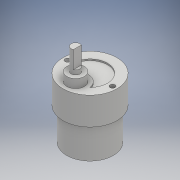
# Autodesk Inventor part: MOTOR DC
Saved by Autodesk Inventor 2018 (Build 220112000, 112)
## iProperties
Created: 2018-03-05
Part Number: MOTOR DC
Material: Generic
Document SubType Name: Modeling
Designer: isai
Density: 1 g/cm^3
Appearance: Default
Author: isai
Autodesk Inventor part; units mm, degrees
ref_plane "YZ Plane" through (0, 0, 0) normal (1, 0, 0) x (0, 1, 0)
ref_plane "XZ Plane" through (0, 0, 0) normal (0, 1, 0) x (-1, 0, 0)
ref_plane "XY Plane" through (0, 0, 0) normal (0, 0, 1) x (1, 0, 0)
sketch "Sketch1" plane through (0, 0, 0) normal (0, 0, 1) x (1, 0, 0)
  circle A0 centre (0, 0) radius 18.5
  line L0 (-15.5, 0) -> (15.5, 0)
  circle A1 centre (-15.5, 0) radius 1.7
  circle A2 centre (15.5, 0) radius 1.7
  dimension "d0" = 37
  dimension "d1" = 31
  dimension "d2" = 3.4
  dimension "d3" = 3.4
  constraints: 4 coincident, 3 centre point, 2 end point, 1 horizontal, 1 midpoint
  measures "d0" diameter of A0
  measures "d1" distance of L0.start L0.end
  measures "d2" diameter of A1
  measures "d3" diameter of A2
extrude "Extrusion1" add sketch "Sketch1" against normal blind 4.5
sketch "Sketch2" plane through (0, 0, 0) normal (0, 0, 1) x (1, 0, 0)
  arc A0 (8.4832, -8.4874) -> (-8.4832, -8.4874) centre (0, -9.9) ccw
  circle A1 centre (0, 0) radius 18.5 projected
  circle A2 centre (0, -9.9) radius 6
  arc A3 (8.4832, -8.4874) -> (-8.4832, -8.4874) centre (0, 0) ccw
  arc A4 (-5.9787, -10.4045) -> (5.9787, -10.4045) centre (0, 0) ccw
  dimension "d10" = 17.2
  dimension "d11" = 12
  constraints: 8 point on circle, 4 centre point, 2 coincident, 1 tangent
  measures "d10" diameter of A0
  measures "d11" diameter of A2
extrude "Extrusion2" add sketch "Sketch2" along normal blind 6 contours A2 A4 | A4 A2
extrude "Extrusion3" cut sketch "Sketch2" against normal blind 1 contours A0 A3
sketch "Sketch3" plane through (0, -9.9, 6) normal (0, 0, 1) x (1, 0, 0)
  circle A0 centre (0, 0) radius 6 projected
  circle A1 centre (0, 0) radius 3
  point P0 (0, 9.9)
  dimension "d16" = 6
  constraints: 1 centre point, 1 coincident
  measures "d16" diameter of A1
extrude "Extrusion4" add sketch "Sketch3" along normal blind 15 contours A1
sketch "Sketch4" plane through (0, 0, -4.5) normal (0, 0, -1) x (-1, 0, 0)
  circle A0 centre (0, 0) radius 18.5 projected
extrude "Extrusion5" add sketch "Sketch4" along normal blind 14.5
sketch "Sketch5" plane through (0, -9.9, 21) normal (0, 0, 1) x (1, 0, 0)
  circle A0 centre (0, 0) radius 3 projected
  line L0 (1.2182, 2.7415) -> (1.2182, -2.7415)
  point P0 (0, 9.9)
  constraints: 2 end point, 2 point on circle, 1 vertical
extrude "Extrusion6" cut sketch "Sketch5" against normal blind 12 contours A0 L0 picked at (1.8121, 0)
sketch "Sketch6" plane through (0, 0, -19) normal (0, 0, -1) x (-1, 0, 0)
  circle A0 centre (0, 0) radius 16
  dimension "d23" = 32
  constraints: 1 centre point, 1 coincident
  measures "d23" diameter of A0
extrude "Extrusion7" add sketch "Sketch6" along normal blind 22
sketch "Sketch7" plane through (0, 0, 0) normal (0, 0, 1) x (1, 0, 0)
  circle A0 centre (-15.5, 0) radius 1.7 projected
  circle A1 centre (15.5, 0) radius 1.7 projected
  circle A2 centre (0, 0) radius 18.5 projected
body "Solid1"
